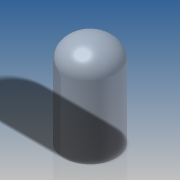
# Autodesk Inventor part: 99961-TransClear
Saved by Autodesk Inventor 2016 SP2 (Build 200236200, 236)
## iProperties
Created: 2015-08-25
Part Number: 99961-TransClear
Material: Polycarbonate
Document SubType Name: Modeling
Designer: D. Kohfeld
Mass: 0.0501851 g
Surface Area: 0.657585 cm^2
Volume: 0.0418209 cm^3
Density: 1.2 g/cm^3
Appearance: TransClear
Author: D. Kohfeld
Autodesk Inventor part; units mm, degrees
ref_plane "YZ Plane" through (0, 0, 0) normal (1, 0, 0) x (0, 1, 0)
ref_plane "XZ Plane" through (0, 0, 0) normal (0, 1, 0) x (-1, 0, 0)
ref_plane "XY Plane" through (0, 0, 0) normal (0, 0, 1) x (1, 0, 0)
sketch "Sketch2" plane through (0, 0, 0) normal (0, 0, 1) x (1, 0, 0)
  line L0 (0, -4.4) -> (0, 1.2)
  line L1 (1.6, 0) -> (1.6, -4.4)
  line L2 (1.6, -4.4) -> (0, -4.4)
  ellipse E0 centre (0, 0) end of major axis (1.6, 0) minor radius 1.2 (1.6, 0) -> (0, 1.2) ccw
  dimension "d2" = 1.2
  dimension "d0" = 3.2
  dimension "d1" = 4.4
  constraints: 6 end point, 3 vertical, 1 coincident, 1 horizontal, 1 point on line, 4 other
  measures "d0" diameter of L1 L0
  measures "d1" distance from line of point (0, 0) L2
revolve "Revolution1" add sketch "Sketch2" angle 360 about axis through (0, -4.4, 0) along (0, 1, 0)
equation "\"d0\" = rd"
equation "\"rd\" = 3.2"
body "Solid1"
